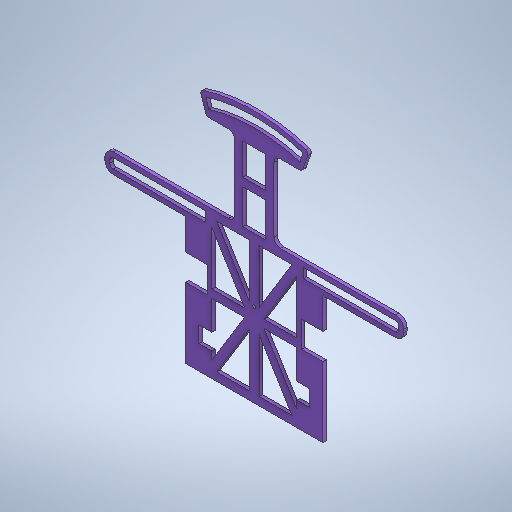
# Autodesk Inventor part: StructureV2Laser
Saved by Autodesk Inventor 2025.1 (Build 291241020, 241B)
## iProperties
Created: 2024-11-23
Part Number: StructureV2Laser
Material: Generic
Document SubType Name: Modeling
Designer: Lucas
Density: 1 g/cm^3
Appearance: Default
Author: Lucas
Autodesk Inventor part; units mm, degrees
ref_plane "YZ Plane" through (0, 0, 0) normal (1, 0, 0) x (0, 1, 0)
ref_plane "XZ Plane" through (0, 0, 0) normal (0, 1, 0) x (-1, 0, 0)
ref_plane "XY Plane" through (0, 0, 0) normal (0, 0, 1) x (1, 0, 0)
sketch "Sketch1" plane through (0, 0, 0) normal (0, 0, 1) x (1, 0, 0)
  line L0 (0, 0) -> (42, 0)
  line L1 (42, 0) -> (42, 90)
  line L2 (42, 90) -> (0, 90)
  line L3 (0, 90) -> (0, 0)
  line L4 (0, 90) -> (16, 90)
  line L5 (16, 90) -> (16, 0)
  line L6 (16, 0) -> (0, 0)
  line L7 (0, 0) -> (0, 90)
  line L8 (16, 90) -> (42, 90)
  line L9 (42, 90) -> (42, 85)
  line L10 (42, 85) -> (16, 85)
  line L11 (16, 85) -> (16, 90)
  line L12 (16, 0) -> (42, 0)
  line L13 (42, 0) -> (42, 5)
  line L14 (42, 5) -> (16, 5)
  line L15 (16, 5) -> (16, 0)
  line L16 (16, 47.5) -> (42, 47.5)
  line L17 (42, 47.5) -> (42, 42.5)
  line L18 (42, 42.5) -> (16, 42.5)
  line L19 (16, 42.5) -> (16, 47.5)
  line L20 (0, 90) -> (-44.5, 90)
  line L21 (-49.5, 85) -> (-49.5, 83)
  line L22 (-44.5, 78) -> (0, 78)
  line L23 (0, 78) -> (0, 90)
  arc A0 (-44.5, 90) -> (-49.5, 85) centre (-44.5, 85) ccw
  arc A1 (-49.5, 83) -> (-44.5, 78) centre (-44.5, 83) ccw
  line L24 (-44.5, 87) -> (-3, 87)
  line L25 (-3, 87) -> (-3, 81)
  line L26 (-3, 81) -> (-44.5, 81)
  arc A2 (-46.5, 83) -> (-44.5, 81) centre (-44.5, 83) ccw
  line L27 (-46.5, 83) -> (-46.5, 85)
  arc A3 (-44.5, 87) -> (-46.5, 85) centre (-44.5, 85) ccw
  line L28 (-3, 87) -> (12, 87)
  line L29 (12, 87) -> (12, 81)
  line L30 (12, 81) -> (-3, 81)
  line L31 (-3, 81) -> (-3, 87)
  line L32 (42, 85) -> (39, 85)
  line L33 (39, 85) -> (39, 5)
  line L34 (39, 5) -> (42, 5)
  line L35 (42, 5) -> (42, 85)
  circle A4 centre (42, 51.037) radius 1
  line L36 (16, 85) -> (39, 47.5) construction
  line L37 (39, 42.5) -> (16, 5) construction
  line L38 (18.9328, 85) -> (39, 52.2817)
  line L39 (36.0672, 47.5) -> (16, 80.2183)
  line L40 (36.0672, 42.5) -> (16, 9.7817)
  line L41 (18.9328, 5) -> (39, 37.7183)
  point P0 (16, 45)
  point P1 (16, 45)
  point P2 (-49.5, 78)
  point P3 (-49.5, 90)
  point P4 (27.5, 23.75)
  point P5 (16, 42.5)
  point P6 (0, 78)
  point P7 (42, 50.037)
  point P8 (42, 52.037)
  dimension "d0" = 42
  dimension "d1" = 90
  dimension "d2" = 16
  dimension "d3" = 5
  dimension "d4" = 26
  dimension "d5" = 5
  dimension "d6" = 26
  dimension "d7" = 5
  dimension "d8" = 49.5
  dimension "d9" = 12
  dimension "d10" = 5
  dimension "d11" = 3
  dimension "d12" = 15
  dimension "d13" = 6
  dimension "d14" = 3
  dimension "d17" = 2
  dimension "d19" = 38.963
  dimension "d20" = 2.5
  dimension "d21" = 2.5
  dimension "d22" = 2.5
  dimension "d23" = 2.5
  constraints: 84 end point, 22 parallel, 21 point on line, 9 perpendicular, 8 horizontal, 8 point on circle, 5 centre point, 4 tangent, 3 midpoint, 1 coincident, 1 equal radius, 5 other
  measures "d0" distance of L2.end L1.end
  measures "d1" distance of L2.end L0.start
  measures "d2" distance of L5.end L6.end
  measures "d3" distance of L8.end L9.end
  measures "d4" distance of L14.end L13.end
  measures "d5" distance of L13.end L12.end
  measures "d6" distance of L17.end L18.end
  measures "d7" distance of L16.end L17.end
  measures "d8" distance of L22.end point (-49.5, 78)
  measures "d9" distance of point (-49.5, 78) point (-49.5, 90)
  measures "d10" radius of A0
  measures "d11" distance between parallel lines of L20 L24
  measures "d12" distance of L29.end L30.end
  measures "d13" distance of L28.end L29.end
  measures "d14" distance of L34.end L33.end
  measures "d17" diameter of A4
  measures "d19" distance from line of L8 A4.centre
  measures "d20" distance between parallel lines of L36 L39
  measures "d21" distance between parallel lines of L38 L36
  measures "d22" distance between parallel lines of L37 L40
  measures "d23" distance from line of point (27.5, 23.75) L41
extrude "Extrusion1" add sketch "Sketch1" along normal blind 2 contours L3 L30 L29 L28 L2 L5 L0 | L5 L14 L1 L0 | L22 A1 L21 A0 L20 L3 L28 L24 A3 L27 A2 L26 L30 | L5 L40 L18 L33 L41 L14 | L14 L33 L18 L1 | L18 L33 L16 L1 | L5 L16 L33 L18 | L16 L33 L10 L1 A4 | L2 L1 L10 L5 | L16 L39 L5 L10 L38 L33
sketch "Sketch2" plane through (0, 0, 2) normal (0, 0, 1) x (1, 0, 0)
  arc A0 (42, 52.037) -> (42, 50.037) centre (42, 51.037) ccw projected
  circle A1 centre (42, 51.037) radius 104 construction
  circle A2 centre (42, 51.037) radius 101 construction
  circle A3 centre (42, 51.037) radius 95 construction
  circle A4 centre (42, 51.037) radius 93 construction
  line L0 (42, 90) -> (-44.5, 90) projected
  line L1 (42, 90) -> (42, -52.963)
  line L2 (42, 155.037) -> (42, 90)
  line L3 (42, 51.037) -> (8.6562, 149.5469) construction
  line L4 (42, 51.037) -> (146, 51.037) construction
  line L5 (42, 51.037) -> (13.2923, 139.4953) construction
  line L6 (42, 51.037) -> (135, 51.037) construction
  line L7 (42, 51.037) -> (12.3019, 147.5721) construction
  line L8 (42, 51.037) -> (143, 51.037) construction
  line L9 (12.3019, 147.5721) -> (14.0662, 141.8373)
  arc A5 (42, 152.037) -> (12.3019, 147.5721) centre (42, 51.037) ccw
  arc A6 (42, 146.037) -> (14.0662, 141.8373) centre (42, 51.037) ccw
  line L10 (14.0662, 141.8373) -> (16.0662, 141.8373) construction
  line L11 (13.2923, 139.4953) -> (13.2923, 137.4953) construction
  line L12 (9.3038, 147.6339) -> (12.2756, 138.8541)
  arc A7 (42, 155.037) -> (10.5942, 150.1817) centre (42, 51.037) ccw
  line L13 (42, 90) -> (30, 90)
  line L14 (30, 94) -> (30, 133.4953)
  line L15 (30, 137.4953) -> (42, 137.4953)
  line L16 (42, 137.4953) -> (42, 90)
  line L17 (14.17, 137.4953) -> (26, 137.4953)
  line L18 (30, 137.4953) -> (35, 137.4953)
  line L19 (35, 137.4953) -> (35, 90)
  line L20 (35, 90) -> (30, 90)
  line L21 (30, 90) -> (30, 137.4953)
  line L22 (35, 137.4953) -> (42, 137.4953)
  line L23 (42, 137.4953) -> (42, 135.4953)
  line L24 (42, 135.4953) -> (35, 135.4953)
  line L25 (35, 135.4953) -> (35, 137.4953)
  line L26 (35, 116.2476) -> (42, 116.2476)
  line L27 (42, 116.2476) -> (42, 111.2476)
  line L28 (42, 111.2476) -> (35, 111.2476)
  line L29 (35, 111.2476) -> (35, 116.2476)
  arc A8 (10.5942, 150.1817) -> (9.3038, 147.6339) centre (11.1982, 148.2751) ccw
  arc A9 (12.2756, 138.8541) -> (14.17, 137.4953) centre (14.17, 139.4953) ccw
  line L30 (26, 90) -> (26, 90)
  arc A10 (26, 90) -> (30, 94) centre (26, 94) ccw
  arc A11 (30, 133.4953) -> (26, 137.4953) centre (26, 133.4953) ccw
  point P0 (0, 0)
  point P1 (12.7355, 137.4953)
  point P2 (35, 113.7476)
  point P3 (35, 113.7476)
  point P4 (42, 152.037)
  dimension "d27" = 202
  dimension "d29" = 186
  dimension "d26" = 208
  dimension "d28" = 190
  dimension "d30" = 108.7
  dimension "d31" = 107.98
  dimension "d32" = 101
  dimension "d33" = 107.1
  dimension "d36" = 2
  dimension "d37" = 12
  dimension "d38" = 5
  dimension "d39" = 2
  dimension "d40" = 7
  dimension "d41" = 5
  dimension "d42" = 2
  dimension "d43" = 2
  dimension "d44" = 4
  dimension "d45" = 4
  constraints: 60 end point, 20 point on circle, 15 point on line, 9 centre point, 9 horizontal, 8 parallel, 8 tangent, 6 perpendicular, 5 coincident, 3 equal length, 2 concentric, 2 midpoint, 1 equal radius, 1 horizontal alignment, 1 vertical, 1 vertical alignment, 6 other
  measures "d26" diameter of A1
  measures "d28" diameter of A3
  measures "d30" angle of L4 L3
  measures "d31" angle of L6 L5
  measures "d32" distance of L3.start L7.end
  measures "d33" angle of L8 L7
  measures "d36" distance of L5.end L11.end
  measures "d37" distance of L15.start L15.end
  measures "d38" distance of L19.end L20.end
  measures "d39" distance of L22.end L23.end
  measures "d40" distance of L27.end L28.end
  measures "d41" distance of L26.end L27.end
  measures "d42" radius of A8
  measures "d43" radius of A9
  measures "d44" distance of L20.end L30.end
  measures "d45" radius of A10
extrude "Extrusion2" add sketch "Sketch2" against normal blind 2 contours L0 L21 L14 L15 L19 | L28 L19 L26 L2 | L0 A10 L21 | L24 L19 L15 L2 | A11 L17 A9 L12 A8 A7 L2 A5 L9 A6 L15 L21
sketch "Sketch3" plane through (0, 0, 2) normal (0, 0, 1) x (1, 0, 0)
  line L0 (0, 59.037) -> (13, 59.037)
  line L1 (13, 59.037) -> (13, 43.037)
  line L2 (13, 43.037) -> (0, 43.037)
  line L3 (0, 43.037) -> (0, 59.037)
  line L4 (12, 81) -> (-44.5, 81) projected
  line L5 (0, 78) -> (0, 0) projected
  line L6 (16, 9.7817) -> (16, 42.5) projected
  line L7 (16, 24.589) -> (8, 24.589)
  line L8 (8, 24.589) -> (8, 14.589)
  line L9 (8, 14.589) -> (16, 14.589)
  line L10 (16, 14.589) -> (16, 24.589)
  line L11 (0, 0) -> (42, 0) projected
  line L12 (26, 90) -> (-44.5, 90) projected
  point P0 (0, 51.037)
  point P1 (16, 19.589)
  dimension "d48" = 13
  dimension "d49" = 16
  dimension "d51" = 0
  dimension "d52" = 8
  dimension "d53" = 10
  dimension "d54" = 19.589
  dimension "d55" = 38.963
  constraints: 16 end point, 4 parallel, 2 horizontal, 2 midpoint, 2 perpendicular, 1 point on line
  measures "d48" distance of L1.end L2.end
  measures "d49" distance of L0.end L1.end
  measures "d51" distance between parallel lines of L5 L3
  measures "d52" distance of L9.end L8.end
  measures "d53" distance of L8.end L7.end
  measures "d54" distance from line of L11 point (16, 19.589)
  measures "d55" distance from line of L12 point (0, 51.037)
extrude "Extrusion3" cut sketch "Sketch3" against normal through all
mirror "Mirror2" about plane through (42, 52.037, 0) normal (1, 0, 0)
body "Solid1"
